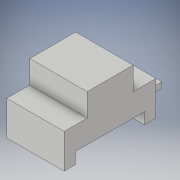
# Autodesk Inventor part: Part1
Saved by Autodesk Inventor 2018 (Build 220112000, 112)
## iProperties
Created: 2020-01-07
Part Number: Part1
Material: Generic
Document SubType Name: Modeling
Designer: AOFUser
Density: 1 g/cm^3
Appearance: Default
Author: AOFUser
Autodesk Inventor part; units mm, degrees
ref_plane "YZ Plane" through (0, 0, 0) normal (1, 0, 0) x (0, 1, 0)
ref_plane "XZ Plane" through (0, 0, 0) normal (0, 1, 0) x (-1, 0, 0)
ref_plane "XY Plane" through (0, 0, 0) normal (0, 0, 1) x (1, 0, 0)
sketch "Sketch1" plane through (0, 0, 0) normal (0, 1, 0) x (-1, 0, 0)
  line L0 (0, 0) -> (-63.5, 0)
  line L1 (-63.5, 0) -> (-63.5, -101.6)
  line L2 (-63.5, -101.6) -> (0, -101.6)
  line L3 (0, -101.6) -> (0, 0)
  dimension "d0" = 63.5
  dimension "d1" = 101.6
  constraints: 8 end point, 2 parallel, 1 horizontal, 1 perpendicular
  measures "d0" distance of L2.end L1.end
  measures "d1" distance of L1.end L0.end
extrude "Extrusion1" add sketch "Sketch1" along normal blind 38.1
sketch "Sketch2" plane through (0, 0, 0) normal (0, -1, 0) x (1, 0, 0)
  line L0 (0, 0) -> (0, -12.7)
  line L1 (0, -101.6) -> (0, 0) projected
  line L2 (63.5, 0) -> (63.5, -101.6) projected
  line L3 (0, -12.7) -> (63.5, -12.7)
  line L4 (63.5, -12.7) -> (63.5, -88.9)
  line L5 (63.5, -88.9) -> (0, -88.9)
  line L6 (0, -88.9) -> (0, -12.7)
  dimension "d4" = 12.7
  dimension "d5" = 76.2
  constraints: 10 end point, 2 parallel, 2 point on line, 1 horizontal, 1 perpendicular
  measures "d4" distance of L0.start L0.end
  measures "d5" distance of L3.end L4.end
extrude "Extrusion2" cut sketch "Sketch2" against normal blind 12.7
sketch "Sketch3" plane through (0, 38.1, 0) normal (0, 1, 0) x (1, 0, 0)
  line L0 (63.5, 0) -> (63.5, 101.6) projected
  line L1 (63.5, 0) -> (63.5, 25.4)
  line L2 (0, 88.9) -> (0, 12.7) projected
  line L3 (63.5, 25.4) -> (0, 25.4)
  line L4 (0, 25.4) -> (0, 76.2)
  line L5 (0, 76.2) -> (63.5, 76.2)
  line L6 (63.5, 76.2) -> (63.5, 25.4)
  point P0 (0, 0)
  dimension "d8" = 25.4
  dimension "d9" = 50.8
  constraints: 10 end point, 2 parallel, 2 point on line, 1 horizontal, 1 perpendicular
  measures "d8" distance of L0.start L1.end
  measures "d9" distance of L3.end L4.end
extrude "Extrusion3" add sketch "Sketch3" along normal blind 25.4
sketch "Sketch4" plane through (63.5, 0, -101.6) normal (0, 0, -1) x (-1, 0, 0)
  line L0 (0, 38.1) -> (0, 63.5) projected
  line L1 (0, 38.1) -> (12.7, 38.1)
  line L2 (63.5, 38.1) -> (0, 38.1) projected
  line L3 (12.7, 38.1) -> (12.7, 19.05)
  line L4 (12.7, 19.05) -> (50.8, 19.05)
  line L5 (50.8, 19.05) -> (50.8, 12.7)
  line L6 (50.8, 12.7) -> (12.7, 12.7)
  line L7 (12.7, 12.7) -> (12.7, 19.05)
  point P0 (63.5, 0)
  dimension "d12" = 12.7
  dimension "d13" = 19.05
  dimension "d14" = 38.1
  dimension "d15" = 6.35
  constraints: 12 end point, 2 parallel, 2 perpendicular, 1 horizontal, 1 point on line
  measures "d12" distance of L0.start L1.end
  measures "d13" distance of L1.end L3.end
  measures "d14" distance of L5.end L6.end
  measures "d15" distance of L4.end L5.end
extrude "Extrusion4" add sketch "Sketch4" along normal blind 19.05
body "Solid1"
